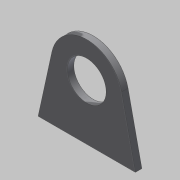
# Autodesk Inventor part: 草圖檔
Saved by Autodesk Inventor 2020 (Build 240168000, 168)
## iProperties
Created: 2015-10-26
Part Number: 草圖檔
Document SubType Name: Modeling
Designer: user
Density: 1 g/cm^3
Material: 一般
Mass: 1.0477 g
Surface Area: 13.2199 cm^2
Volume: 1.0477 cm^3
Appearance: 預設
Author: user
Autodesk Inventor part; units mm, degrees
ref_plane "YZ Plane" through (0, 0, 0) normal (1, 0, 0) x (0, 1, 0)
ref_plane "XZ Plane" through (0, 0, 0) normal (0, 1, 0) x (-1, 0, 0)
ref_plane "XY Plane" through (0, 0, 0) normal (0, 0, 1) x (1, 0, 0)
sketch "草圖2" plane through (0, 0, 0) normal (0, 1, 0) x (-1, 0, 0)
  line L0 (0, 0) -> (25, 0) construction
  line L1 (0, 0) -> (0, 21.0714) construction
  line L2 (-15, 0) -> (15, 0)
  line L3 (15, 0) -> (10.7434, 19.3619)
  line L4 (-10.7434, 19.3619) -> (-15, 0)
  arc A0 (10.7434, 19.3619) -> (-10.7434, 19.3619) centre (0, 17) ccw
  circle A1 centre (0, 17) radius 6
  dimension "d4" = 12
  dimension "d10" = 30
  dimension "d11" = 17
  dimension "d12" = 5
  constraints: 10 end point, 2 centre point, 2 horizontal, 2 point on circle, 2 tangent, 1 coincident, 1 midpoint, 1 perpendicular, 1 other
  measures "d4" diameter of A1
  measures "d10" distance of L2.start L2.end
  measures "d11" distance from line of A0.centre L2
  measures "d12" radial gap between concentric circles of A1 A0
extrude "擠出1" add sketch "草圖2" along normal mid plane 2
